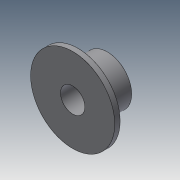
# Autodesk Inventor part: HEDR-5420-ES214_DISC
Saved by Autodesk Inventor 2018.3 (Build 223284000, 284)
## iProperties
Created: 2018-12-16
Material: Generic
Vendor: HHMI: JRC - ID&F
Document SubType Name: Modeling
Designer: arnoldj
Density: 1 g/cm^3
Appearance: Default
RuleStatus: InUse
AfterDocSave0: file://Part Number Cleaner
DESIGN DEPARTMENT: HHMI: JRC - ID&F
ALTERED ITEM PART NUMBER: N/A
ALTERED ITEM VENDOR: N/A
ALTERED ITEM DESCRIPTION: N/A
Author: arnoldj
Revision Number: 0
Autodesk Inventor part; units mm, degrees
ref_plane "YZ Plane" through (0, 0, 0) normal (1, 0, 0) x (0, 1, 0)
ref_plane "XZ Plane" through (0, 0, 0) normal (0, 1, 0) x (-1, 0, 0)
ref_plane "XY Plane" through (0, 0, 0) normal (0, 0, 1) x (1, 0, 0)
sketch "Sketch1" plane through (0, 0, 0) normal (0, 0, 1) x (1, 0, 0)
  line L0 (0, 7) -> (0, -7) projected
  line L1 (-7, 0) -> (7, 0) projected
  circle A0 centre (0, 0) radius 5
  circle A1 centre (0, 0) radius 2.5
  dimension "d0" = 10
  dimension "d1" = 5
  constraints: 2 centre point, 2 coincident
  measures "d0" diameter of A0
  measures "d1" diameter of A1
extrude "Extrusion1" add sketch "Sketch1" along normal blind 6 contours A0 L1 A1 L0 | L0 A1 L1 A0 | A0 L0 A1 L1 | L1 A1 L0 A0
sketch "Sketch2" plane through (0, 0, 6) normal (0, 0, 1) x (1, 0, 0)
  circle A0 centre (0, 0) radius 2.5 projected
  circle A1 centre (0, 0) radius 5 projected
  circle A2 centre (0, 0) radius 8.625
  dimension "d4" = 17.25
  constraints: 1 centre point, 1 coincident
  measures "d4" diameter of A2
extrude "Extrusion2" add sketch "Sketch2" along normal blind 1.1 contours A1 | A2
sketch "Sketch3" plane through (0, 0, 0) normal (1, 0, 0) x (0, 1, 0)
  line L0 (0, 8.52) -> (0, -1.42) projected
  line L1 (-12.075, 0) -> (12.075, 0) projected
  point P0 (0, 0)
  point P1 (0, 2)
  dimension "d7" = 2
  constraints: 1 point on line
  measures "d7" distance from line of L1 point (0, 2)
hole "Hole1" at (0, 0, 2) direction (-1, 0, 0) diameter 2.4638 end through all
body "Solid1"
